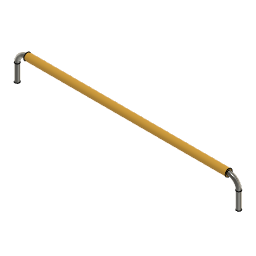
Full Piano (Autodesk Fusion 360 archive; units mm, degrees)
design "Yellow 13"
Autodesk Fusion 360 part; units mm, degrees
sketch "Sketch1" plane through (0, 0, 0) normal (0, 1, 0) x (1, 0, 0)
  line L0 (1.5, 0) -> (31.52, 0)
  line L1 (0, 1.5) -> (0, 4)
  line L2 (33.02, 1.5) -> (33.02, 4)
  arc A0 (0, 1.5) -> (1.5, 0) centre (1.5, 1.5) ccw
  arc A1 (31.52, 0) -> (33.02, 1.5) centre (31.52, 1.5) ccw
  point P0 (33.02, 0)
  dimension "d6" = 33.02
  dimension "d7" = 4
  dimension "d8" = 4
  dimension "d10" = 1.5
  dimension "d11" = 1.5
  constraint horizontal L0
  constraint perpendicular L0 L1
  constraint perpendicular L0 L2
  constraint coincident origin L0
  constraint coincident origin L1
  constraint tangent L1 A0
  constraint tangent L0 A0
  constraint coincident P0 L0
  constraint coincident P0 L2
  constraint tangent L0 A1
  constraint tangent L2 A1
  measures "d6" distance of origin P0
  measures "d7" distance of origin L1.end
  measures "d8" distance of P0 L2.end
  measures "d10" radius of A0
  measures "d11" radius of A1
pipe "Pipe1" add diameter 0.64 path "Sketch1" along L1 A0 L0 A1 L2 makes body 1
ref_plane "WorkPlane1" through (1.5, 0, 0) normal (1, 0, 0) x (0, 1, 0)
sketch "Sketch2" plane through (1.5, 0, 0) normal (1, 0, 0) x (0, 1, 0)
  circle A0 centre (0, 0) radius 0.52
  circle A1 centre (0, 0) radius 0.32
  dimension "d18" = 1.04
  dimension "d19" = 0.64
  constraint coincident A0.centre A1.centre
  constraint concentric A0 A1
  measures "d18" diameter of A0
  measures "d19" diameter of A1
ref_plane "WorkPlane2" through (31.52, 0, 0) normal (1, 0, 0) x (0, 1, 0)
extrude "Extrude1" add sketch "Sketch2" along normal up to surface (30.02 mm away) separate body makes body 2
equation "WireGauge = 0.64 mm"
equation "InsulationThickness = 0.4 mm"
equation "Length = 13"
equation "HoleSpacing = 2.54 mm"
equation "d6 = HoleSpacing * Length"
equation "d7 = ExtraLength"
equation "d8 = ExtraLength"
equation "ExtraLength = 4 mm"
equation "d10 = Arc"
equation "d11 = Arc"
equation "Arc = 1.5 mm"
equation "d15 = WireGauge"
equation "d18 = InsulationThickness + WireGauge"
equation "d19 = WireGauge"

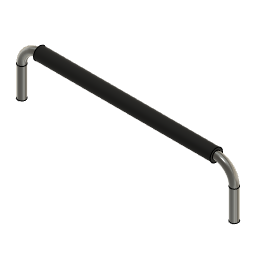
design "Black 8"
Autodesk Fusion 360 part; units mm, degrees
sketch "Sketch1" plane through (0, 0, 0) normal (0, 1, 0) x (1, 0, 0)
  line L0 (1.5, 0) -> (16.28, 0)
  line L1 (0, 1.5) -> (0, 4)
  line L2 (17.78, 1.5) -> (17.78, 4)
  arc A0 (0, 1.5) -> (1.5, 0) centre (1.5, 1.5) ccw
  arc A1 (16.28, 0) -> (17.78, 1.5) centre (16.28, 1.5) ccw
  point P0 (17.78, 0)
  dimension "d6" = 17.78
  dimension "d7" = 4
  dimension "d8" = 4
  dimension "d10" = 1.5
  dimension "d11" = 1.5
  constraint horizontal L0
  constraint perpendicular L0 L1
  constraint perpendicular L0 L2
  constraint coincident origin L0
  constraint coincident origin L1
  constraint tangent L1 A0
  constraint tangent L0 A0
  constraint coincident P0 L0
  constraint coincident P0 L2
  constraint tangent L0 A1
  constraint tangent L2 A1
  measures "d6" distance of origin P0
  measures "d7" distance of origin L1.end
  measures "d8" distance of P0 L2.end
  measures "d10" radius of A0
  measures "d11" radius of A1
pipe "Pipe1" add diameter 0.64 path "Sketch1" along L1 A0 L0 A1 L2 makes body 1
ref_plane "WorkPlane1" through (1.5, 0, 0) normal (1, 0, 0) x (0, 1, 0)
sketch "Sketch2" plane through (1.5, 0, 0) normal (1, 0, 0) x (0, 1, 0)
  circle A0 centre (0, 0) radius 0.52
  circle A1 centre (0, 0) radius 0.32
  dimension "d18" = 1.04
  dimension "d19" = 0.64
  constraint coincident A0.centre A1.centre
  constraint concentric A0 A1
  measures "d18" diameter of A0
  measures "d19" diameter of A1
ref_plane "WorkPlane2" through (16.28, 0, 0) normal (1, 0, 0) x (0, 1, 0)
extrude "Extrude1" add sketch "Sketch2" along normal up to surface (14.78 mm away) separate body makes body 2
equation "WireGauge = 0.64 mm"
equation "InsulationThickness = 0.4 mm"
equation "Length = 8"
equation "HoleSpacing = 2.54 mm"
equation "d6 = HoleSpacing * ( Length - 1 )"
equation "d7 = ExtraLength"
equation "d8 = ExtraLength"
equation "ExtraLength = 4 mm"
equation "d10 = Arc"
equation "d11 = Arc"
equation "Arc = 1.5 mm"
equation "d15 = WireGauge"
equation "d18 = InsulationThickness + WireGauge"
equation "d19 = WireGauge"

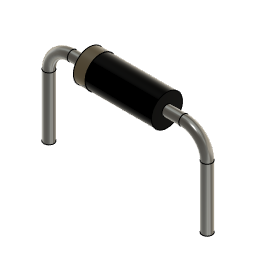
design "Diode 2"
Autodesk Fusion 360 part; units mm, degrees
sketch "Sketch1" plane through (0, 0, 0) normal (0, 1, 0) x (1, 0, 0)
  line L0 (1.5, 0) -> (8.66, 0)
  line L1 (0, 1.5) -> (0, 5.5)
  line L2 (10.16, 1.5) -> (10.16, 5.5)
  arc A0 (0, 1.5) -> (1.5, 0) centre (1.5, 1.5) ccw
  arc A1 (8.66, 0) -> (10.16, 1.5) centre (8.66, 1.5) ccw
  point P0 (10.16, 0)
  dimension "d6" = 10.16
  dimension "d7" = 5.5
  dimension "d8" = 5.5
  dimension "d10" = 1.5
  dimension "d11" = 1.5
  constraint horizontal L0
  constraint perpendicular L0 L1
  constraint perpendicular L0 L2
  constraint coincident origin L0
  constraint coincident origin L1
  constraint tangent L1 A0
  constraint tangent L0 A0
  constraint coincident P0 L0
  constraint coincident P0 L2
  constraint tangent L0 A1
  constraint tangent L2 A1
  measures "d6" distance of origin P0
  measures "d7" distance of origin L1.end
  measures "d8" distance of P0 L2.end
  measures "d10" radius of A0
  measures "d11" radius of A1
pipe "Pipe1" add diameter 0.64 path "Sketch1" along L1 A0 L0 A1 L2
ref_plane "WorkPlane1" through (1.5, 0, 0) normal (1, 0, 0) x (0, 1, 0)
sketch "Sketch2" plane through (1.5, 0, 0) normal (1, 0, 0) x (0, 1, 0)
  circle A0 centre (0, 0) radius 0.52
  circle A1 centre (0, 0) radius 0.32
  dimension "d18" = 1.04
  dimension "d19" = 0.64
  constraint coincident A0.centre A1.centre
  constraint concentric A0 A1
  measures "d18" diameter of A0
  measures "d19" diameter of A1
ref_plane "WorkPlane2" through (8.66, 0, 0) normal (1, 0, 0) x (0, 1, 0)
ref_plane "WorkPlane3" through (-0.32, 0, -3.8241) normal (-1, 0, 0) x (0, 1, 0)
ref_plane "WorkPlane4" through (10.48, 0, -1.931) normal (1, 0, 0) x (0, 1, 0)
ref_plane "WorkPlane5" through (5.08, 0, -3.8241) normal (-1, 0, 0) x (0, 1, 0)
sketch "Sketch3" plane through (5.08, 0, -2.3241) normal (-1, 0, 0) x (0, 1, 0)
  circle A0 centre (0, -2.3241) radius 0.32
  circle A1 centre (0, -2.3241) radius 1
  dimension "d27" = 2
  constraint concentric A0 A1
  measures "d27" diameter of A1
extrude "Extrude2" add sketch "Sketch3" along normal mid plane 5
sketch "Sketch4" plane through (2.58, 0, 0) normal (-1, 0, 0) x (0, -1, 0)
  circle A0 centre (0, 0) radius 0.32
  circle A1 centre (0, 0) radius 1
  circle A2 centre (0, 0) radius 1.01
  dimension "d30" = 0.01
  constraint coincident A0.centre A1.centre
  measures "d30" distance of A1 A2
extrude "Extrude3" add sketch "Sketch4" against normal blind 0.75 contours A2
equation "WireGauge = 0.64 mm"
equation "InsulationThickness = 0.4 mm"
equation "Length = 5"
equation "HoleSpacing = 2.54 mm"
equation "d6 = HoleSpacing * ( Length - 1 )"
equation "d7 = ExtraLength"
equation "d8 = ExtraLength"
equation "ExtraLength = 5.5 mm"
equation "d10 = Arc"
equation "d11 = Arc"
equation "Arc = 1.5 mm"
equation "d15 = WireGauge"
equation "d18 = InsulationThickness + WireGauge"
equation "d19 = WireGauge"

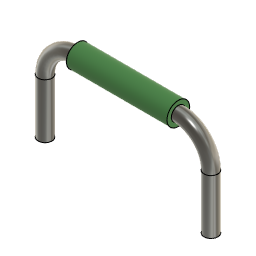
design "Green 4"
Autodesk Fusion 360 part; units mm, degrees
sketch "Sketch1" plane through (0, 0, 0) normal (0, 1, 0) x (1, 0, 0)
  line L0 (1.5, 0) -> (6.12, 0)
  line L1 (0, 1.5) -> (0, 4)
  line L2 (7.62, 1.5) -> (7.62, 4)
  arc A0 (0, 1.5) -> (1.5, 0) centre (1.5, 1.5) ccw
  arc A1 (6.12, 0) -> (7.62, 1.5) centre (6.12, 1.5) ccw
  point P0 (7.62, 0)
  dimension "d6" = 7.62
  dimension "d7" = 4
  dimension "d8" = 4
  dimension "d10" = 1.5
  dimension "d11" = 1.5
  constraint horizontal L0
  constraint perpendicular L0 L1
  constraint perpendicular L0 L2
  constraint coincident origin L0
  constraint coincident origin L1
  constraint tangent L1 A0
  constraint tangent L0 A0
  constraint coincident P0 L0
  constraint coincident P0 L2
  constraint tangent L0 A1
  constraint tangent L2 A1
  measures "d6" distance of origin P0
  measures "d7" distance of origin L1.end
  measures "d8" distance of P0 L2.end
  measures "d10" radius of A0
  measures "d11" radius of A1
pipe "Pipe1" add diameter 0.64 path "Sketch1" along L1 A0 L0 A1 L2 makes body 1
ref_plane "WorkPlane1" through (1.5, 0, 0) normal (1, 0, 0) x (0, 1, 0)
sketch "Sketch2" plane through (1.5, 0, 0) normal (1, 0, 0) x (0, 1, 0)
  circle A0 centre (0, 0) radius 0.52
  circle A1 centre (0, 0) radius 0.32
  dimension "d18" = 1.04
  dimension "d19" = 0.64
  constraint coincident A0.centre A1.centre
  constraint concentric A0 A1
  measures "d18" diameter of A0
  measures "d19" diameter of A1
ref_plane "WorkPlane2" through (6.12, 0, 0) normal (1, 0, 0) x (0, 1, 0)
extrude "Extrude1" add sketch "Sketch2" along normal up to surface (4.62 mm away) separate body makes body 2
equation "WireGauge = 0.64 mm"
equation "InsulationThickness = 0.4 mm"
equation "Length = 4"
equation "HoleSpacing = 2.54 mm"
equation "d6 = HoleSpacing * ( Length - 1 )"
equation "d7 = ExtraLength"
equation "d8 = ExtraLength"
equation "ExtraLength = 4 mm"
equation "d10 = Arc"
equation "d11 = Arc"
equation "Arc = 1.5 mm"
equation "d15 = WireGauge"
equation "d18 = InsulationThickness + WireGauge"
equation "d19 = WireGauge"

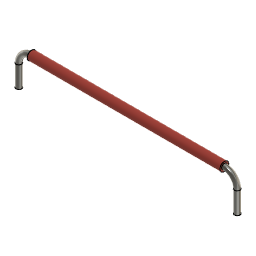
design "Red Diagonal"
Autodesk Fusion 360 part; units mm, degrees
sketch "Sketch1" plane through (0, 0, 0) normal (0, 1, 0) x (1, 0, 0)
  line L0 (1.5, 0) -> (24.0267, 0)
  line L1 (0, 1.5) -> (0, 4)
  line L2 (25.5267, 1.5) -> (25.5267, 4)
  arc A0 (0, 1.5) -> (1.5, 0) centre (1.5, 1.5) ccw
  arc A1 (24.0267, 0) -> (25.5267, 1.5) centre (24.0267, 1.5) ccw
  point P0 (25.5267, 0)
  dimension "d6" = 25.5267
  dimension "d7" = 4
  dimension "d8" = 4
  dimension "d10" = 1.5
  dimension "d11" = 1.5
  constraint horizontal L0
  constraint perpendicular L0 L1
  constraint perpendicular L0 L2
  constraint coincident origin L0
  constraint coincident origin L1
  constraint tangent L1 A0
  constraint tangent L0 A0
  constraint coincident P0 L0
  constraint coincident P0 L2
  constraint tangent L0 A1
  constraint tangent L2 A1
  measures "d6" distance of origin P0
  measures "d7" distance of origin L1.end
  measures "d8" distance of P0 L2.end
  measures "d10" radius of A0
  measures "d11" radius of A1
pipe "Pipe1" add diameter 0.64 path "Sketch1" along L1 A0 L0 A1 L2 makes body 1
ref_plane "WorkPlane1" through (1.5, 0, 0) normal (1, 0, 0) x (0, 1, 0)
sketch "Sketch2" plane through (1.5, 0, 0) normal (1, 0, 0) x (0, 1, 0)
  circle A0 centre (0, 0) radius 0.52
  circle A1 centre (0, 0) radius 0.32
  dimension "d18" = 1.04
  dimension "d19" = 0.64
  constraint coincident A0.centre A1.centre
  constraint concentric A0 A1
  measures "d18" diameter of A0
  measures "d19" diameter of A1
ref_plane "WorkPlane2" through (24.0267, 0, 0) normal (1, 0, 0) x (0, 1, 0)
extrude "Extrude1" add sketch "Sketch2" along normal up to surface (22.5267 mm away) separate body makes body 2
equation "WireGauge = 0.64 mm"
equation "InsulationThickness = 0.4 mm"
equation "Length = 4"
equation "HoleSpacing = 2.54 mm"
equation "d7 = ExtraLength"
equation "d8 = ExtraLength"
equation "ExtraLength = 4 mm"
equation "d10 = Arc"
equation "d11 = Arc"
equation "Arc = 1.5 mm"
equation "d15 = WireGauge"
equation "d18 = InsulationThickness + WireGauge"
equation "d19 = WireGauge"

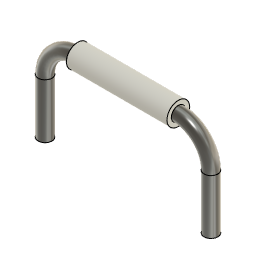
design "White 4"
Autodesk Fusion 360 part; units mm, degrees
sketch "Sketch1" plane through (0, 0, 0) normal (0, 1, 0) x (1, 0, 0)
  line L0 (1.5, 0) -> (6.12, 0)
  line L1 (0, 1.5) -> (0, 4)
  line L2 (7.62, 1.5) -> (7.62, 4)
  arc A0 (0, 1.5) -> (1.5, 0) centre (1.5, 1.5) ccw
  arc A1 (6.12, 0) -> (7.62, 1.5) centre (6.12, 1.5) ccw
  point P0 (7.62, 0)
  dimension "d6" = 7.62
  dimension "d7" = 4
  dimension "d8" = 4
  dimension "d10" = 1.5
  dimension "d11" = 1.5
  constraint horizontal L0
  constraint perpendicular L0 L1
  constraint perpendicular L0 L2
  constraint coincident origin L0
  constraint coincident origin L1
  constraint tangent L1 A0
  constraint tangent L0 A0
  constraint coincident P0 L0
  constraint coincident P0 L2
  constraint tangent L0 A1
  constraint tangent L2 A1
  measures "d6" distance of origin P0
  measures "d7" distance of origin L1.end
  measures "d8" distance of P0 L2.end
  measures "d10" radius of A0
  measures "d11" radius of A1
pipe "Pipe1" add diameter 0.64 path "Sketch1" along L1 A0 L0 A1 L2 makes body 1
ref_plane "WorkPlane1" through (1.5, 0, 0) normal (1, 0, 0) x (0, 1, 0)
sketch "Sketch2" plane through (1.5, 0, 0) normal (1, 0, 0) x (0, 1, 0)
  circle A0 centre (0, 0) radius 0.52
  circle A1 centre (0, 0) radius 0.32
  dimension "d18" = 1.04
  dimension "d19" = 0.64
  constraint coincident A0.centre A1.centre
  constraint concentric A0 A1
  measures "d18" diameter of A0
  measures "d19" diameter of A1
ref_plane "WorkPlane2" through (6.12, 0, 0) normal (1, 0, 0) x (0, 1, 0)
extrude "Extrude1" add sketch "Sketch2" along normal up to surface (4.62 mm away) separate body makes body 2
equation "WireGauge = 0.64 mm"
equation "InsulationThickness = 0.4 mm"
equation "Length = 4"
equation "HoleSpacing = 2.54 mm"
equation "d6 = HoleSpacing * ( Length - 1 )"
equation "d7 = ExtraLength"
equation "d8 = ExtraLength"
equation "ExtraLength = 4 mm"
equation "d10 = Arc"
equation "d11 = Arc"
equation "Arc = 1.5 mm"
equation "d15 = WireGauge"
equation "d18 = InsulationThickness + WireGauge"
equation "d19 = WireGauge"

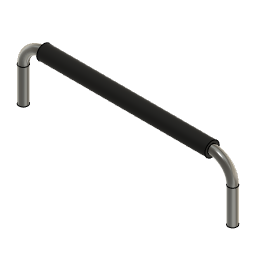
design "Black 7"
Autodesk Fusion 360 part; units mm, degrees
sketch "Sketch1" plane through (0, 0, 0) normal (0, 1, 0) x (1, 0, 0)
  line L0 (1.5, 0) -> (13.74, 0)
  line L1 (0, 1.5) -> (0, 4)
  line L2 (15.24, 1.5) -> (15.24, 4)
  arc A0 (0, 1.5) -> (1.5, 0) centre (1.5, 1.5) ccw
  arc A1 (13.74, 0) -> (15.24, 1.5) centre (13.74, 1.5) ccw
  point P0 (15.24, 0)
  dimension "d6" = 15.24
  dimension "d7" = 4
  dimension "d8" = 4
  dimension "d10" = 1.5
  dimension "d11" = 1.5
  constraint horizontal L0
  constraint perpendicular L0 L1
  constraint perpendicular L0 L2
  constraint coincident origin L0
  constraint coincident origin L1
  constraint tangent L1 A0
  constraint tangent L0 A0
  constraint coincident P0 L0
  constraint coincident P0 L2
  constraint tangent L0 A1
  constraint tangent L2 A1
  measures "d6" distance of origin P0
  measures "d7" distance of origin L1.end
  measures "d8" distance of P0 L2.end
  measures "d10" radius of A0
  measures "d11" radius of A1
pipe "Pipe1" add diameter 0.64 path "Sketch1" along L1 A0 L0 A1 L2 makes body 1
ref_plane "WorkPlane1" through (1.5, 0, 0) normal (1, 0, 0) x (0, 1, 0)
sketch "Sketch2" plane through (1.5, 0, 0) normal (1, 0, 0) x (0, 1, 0)
  circle A0 centre (0, 0) radius 0.52
  circle A1 centre (0, 0) radius 0.32
  dimension "d18" = 1.04
  dimension "d19" = 0.64
  constraint coincident A0.centre A1.centre
  constraint concentric A0 A1
  measures "d18" diameter of A0
  measures "d19" diameter of A1
ref_plane "WorkPlane2" through (13.74, 0, 0) normal (1, 0, 0) x (0, 1, 0)
extrude "Extrude1" add sketch "Sketch2" along normal up to surface (12.24 mm away) separate body makes body 2
equation "WireGauge = 0.64 mm"
equation "InsulationThickness = 0.4 mm"
equation "Length = 7"
equation "HoleSpacing = 2.54 mm"
equation "d6 = HoleSpacing * ( Length - 1 )"
equation "d7 = ExtraLength"
equation "d8 = ExtraLength"
equation "ExtraLength = 4 mm"
equation "d10 = Arc"
equation "d11 = Arc"
equation "Arc = 1.5 mm"
equation "d15 = WireGauge"
equation "d18 = InsulationThickness + WireGauge"
equation "d19 = WireGauge"

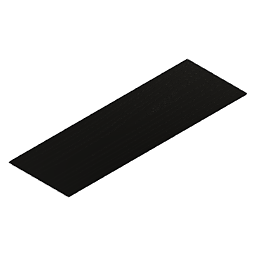
design "Piano Small Key"
Autodesk Fusion 360 part; units mm, degrees
sketch "Sketch1" plane through (0, 0, 0) normal (0, 0, 1) x (1, 0, 0)
  line L0 (0, 0) -> (152.4, 0)
  line L1 (152.4, 0) -> (152.4, 457.2)
  line L2 (152.4, 457.2) -> (0, 457.2)
  line L3 (0, 457.2) -> (0, 0)
  dimension "d4" = 152.4
  dimension "d5" = 457.2
  constraint horizontal L0
  constraint vertical L1
  constraint horizontal L2
  constraint vertical L3
  constraint coincident L0.start L3.end
  measures "d4" distance of L1.end L2.end
  measures "d5" distance of L0.start L2.end
extrude "Extrude1" add sketch "Sketch1" along normal blind 1
equation "SmallKeyWidth = 5.75 in"
equation "SmallKeyHeight = 18 in"
equation "d5 = SmallKeyHeight"

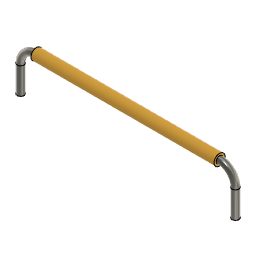
design "Yellow 8"
Autodesk Fusion 360 part; units mm, degrees
sketch "Sketch1" plane through (0, 0, 0) normal (0, 1, 0) x (1, 0, 0)
  line L0 (1.5, 0) -> (18.82, 0)
  line L1 (0, 1.5) -> (0, 4)
  line L2 (20.32, 1.5) -> (20.32, 4)
  arc A0 (0, 1.5) -> (1.5, 0) centre (1.5, 1.5) ccw
  arc A1 (18.82, 0) -> (20.32, 1.5) centre (18.82, 1.5) ccw
  point P0 (20.32, 0)
  dimension "d6" = 20.32
  dimension "d7" = 4
  dimension "d8" = 4
  dimension "d10" = 1.5
  dimension "d11" = 1.5
  constraint horizontal L0
  constraint perpendicular L0 L1
  constraint perpendicular L0 L2
  constraint coincident origin L0
  constraint coincident origin L1
  constraint tangent L1 A0
  constraint tangent L0 A0
  constraint coincident P0 L0
  constraint coincident P0 L2
  constraint tangent L0 A1
  constraint tangent L2 A1
  measures "d6" distance of origin P0
  measures "d7" distance of origin L1.end
  measures "d8" distance of P0 L2.end
  measures "d10" radius of A0
  measures "d11" radius of A1
pipe "Pipe1" add diameter 0.64 path "Sketch1" along L1 A0 L0 A1 L2 makes body 1
ref_plane "WorkPlane1" through (1.5, 0, 0) normal (1, 0, 0) x (0, 1, 0)
sketch "Sketch2" plane through (1.5, 0, 0) normal (1, 0, 0) x (0, 1, 0)
  circle A0 centre (0, 0) radius 0.52
  circle A1 centre (0, 0) radius 0.32
  dimension "d18" = 1.04
  dimension "d19" = 0.64
  constraint coincident A0.centre A1.centre
  constraint concentric A0 A1
  measures "d18" diameter of A0
  measures "d19" diameter of A1
ref_plane "WorkPlane2" through (18.82, 0, 0) normal (1, 0, 0) x (0, 1, 0)
extrude "Extrude1" add sketch "Sketch2" along normal up to surface (17.32 mm away) separate body makes body 2
equation "WireGauge = 0.64 mm"
equation "InsulationThickness = 0.4 mm"
equation "Length = 8"
equation "HoleSpacing = 2.54 mm"
equation "d6 = HoleSpacing * Length"
equation "d7 = ExtraLength"
equation "d8 = ExtraLength"
equation "ExtraLength = 4 mm"
equation "d10 = Arc"
equation "d11 = Arc"
equation "Arc = 1.5 mm"
equation "d15 = WireGauge"
equation "d18 = InsulationThickness + WireGauge"
equation "d19 = WireGauge"

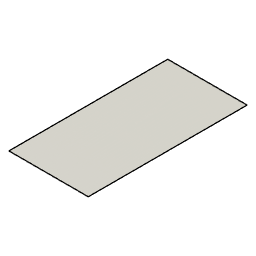
design "Piano Key Full"
Autodesk Fusion 360 part; units mm, degrees
sketch "Sketch1" plane through (0, 0, 0) normal (0, 0, 1) x (1, 0, 0)
  line L0 (0, 0) -> (304.8, 0)
  line L1 (304.8, 0) -> (304.8, 609.6)
  line L2 (304.8, 609.6) -> (0, 609.6)
  line L3 (0, 609.6) -> (0, 0)
  line L4 (0, 609.6) -> (146.05, 609.6)
  line L5 (0, 152.4) -> (0, 609.6)
  dimension "d1" = 304.8
  dimension "d2" = 609.6
  constraint horizontal L0
  constraint vertical L1
  constraint horizontal L2
  constraint vertical L3
  constraint coincident L0.start L3.end
  constraint horizontal L4
  constraint vertical L5
  measures "d1" distance of L1.end L2.end
  measures "d2" distance of L0.start L2.end
extrude "Extrude1" add sketch "Sketch1" along normal blind 1
equation "d1 = KeyWidth"
equation "d2 = KeyHeight"
equation "KeyWidth = 12 in"
equation "KeyHeight = 24 in"
equation "SmallKeyWidth = 5.75 in"
equation "SmallKeyHeight = 18 in"

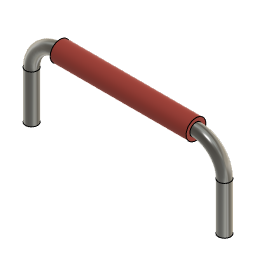
design "Red 5"
Autodesk Fusion 360 part; units mm, degrees
sketch "Sketch1" plane through (0, 0, 0) normal (0, 1, 0) x (1, 0, 0)
  line L0 (1.5, 0) -> (8.66, 0)
  line L1 (0, 1.5) -> (0, 4)
  line L2 (10.16, 1.5) -> (10.16, 4)
  arc A0 (0, 1.5) -> (1.5, 0) centre (1.5, 1.5) ccw
  arc A1 (8.66, 0) -> (10.16, 1.5) centre (8.66, 1.5) ccw
  point P0 (10.16, 0)
  dimension "d6" = 10.16
  dimension "d7" = 4
  dimension "d8" = 4
  dimension "d10" = 1.5
  dimension "d11" = 1.5
  constraint horizontal L0
  constraint perpendicular L0 L1
  constraint perpendicular L0 L2
  constraint coincident origin L0
  constraint coincident origin L1
  constraint tangent L1 A0
  constraint tangent L0 A0
  constraint coincident P0 L0
  constraint coincident P0 L2
  constraint tangent L0 A1
  constraint tangent L2 A1
  measures "d6" distance of origin P0
  measures "d7" distance of origin L1.end
  measures "d8" distance of P0 L2.end
  measures "d10" radius of A0
  measures "d11" radius of A1
pipe "Pipe1" add diameter 0.64 path "Sketch1" along L1 A0 L0 A1 L2 makes body 1
ref_plane "WorkPlane1" through (1.5, 0, 0) normal (1, 0, 0) x (0, 1, 0)
sketch "Sketch2" plane through (1.5, 0, 0) normal (1, 0, 0) x (0, 1, 0)
  circle A0 centre (0, 0) radius 0.52
  circle A1 centre (0, 0) radius 0.32
  dimension "d18" = 1.04
  dimension "d19" = 0.64
  constraint coincident A0.centre A1.centre
  constraint concentric A0 A1
  measures "d18" diameter of A0
  measures "d19" diameter of A1
ref_plane "WorkPlane2" through (8.66, 0, 0) normal (1, 0, 0) x (0, 1, 0)
extrude "Extrude1" add sketch "Sketch2" along normal up to surface (7.16 mm away) separate body makes body 2
equation "WireGauge = 0.64 mm"
equation "InsulationThickness = 0.4 mm"
equation "Length = 5"
equation "HoleSpacing = 2.54 mm"
equation "d6 = HoleSpacing * ( Length - 1 )"
equation "d7 = ExtraLength"
equation "d8 = ExtraLength"
equation "ExtraLength = 4 mm"
equation "d10 = Arc"
equation "d11 = Arc"
equation "Arc = 1.5 mm"
equation "d15 = WireGauge"
equation "d18 = InsulationThickness + WireGauge"
equation "d19 = WireGauge"

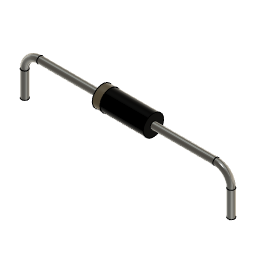
design "Diode 1"
Autodesk Fusion 360 part; units mm, degrees
sketch "Sketch1" plane through (0, 0, 0) normal (0, 1, 0) x (1, 0, 0)
  line L0 (1.5, 0) -> (18.82, 0)
  line L1 (0, 1.5) -> (0, 4)
  line L2 (20.32, 1.5) -> (20.32, 4)
  arc A0 (0, 1.5) -> (1.5, 0) centre (1.5, 1.5) ccw
  arc A1 (18.82, 0) -> (20.32, 1.5) centre (18.82, 1.5) ccw
  point P0 (20.32, 0)
  dimension "d6" = 20.32
  dimension "d7" = 4
  dimension "d8" = 4
  dimension "d10" = 1.5
  dimension "d11" = 1.5
  constraint horizontal L0
  constraint perpendicular L0 L1
  constraint perpendicular L0 L2
  constraint coincident origin L0
  constraint coincident origin L1
  constraint tangent L1 A0
  constraint tangent L0 A0
  constraint coincident P0 L0
  constraint coincident P0 L2
  constraint tangent L0 A1
  constraint tangent L2 A1
  measures "d6" distance of origin P0
  measures "d7" distance of origin L1.end
  measures "d8" distance of P0 L2.end
  measures "d10" radius of A0
  measures "d11" radius of A1
pipe "Pipe1" add diameter 0.64 path "Sketch1" along L1 A0 L0 A1 L2
ref_plane "WorkPlane1" through (1.5, 0, 0) normal (1, 0, 0) x (0, 1, 0)
sketch "Sketch2" plane through (1.5, 0, 0) normal (1, 0, 0) x (0, 1, 0)
  circle A0 centre (0, 0) radius 0.52
  circle A1 centre (0, 0) radius 0.32
  dimension "d18" = 1.04
  dimension "d19" = 0.64
  constraint coincident A0.centre A1.centre
  constraint concentric A0 A1
  measures "d18" diameter of A0
  measures "d19" diameter of A1
ref_plane "WorkPlane2" through (18.82, 0, 0) normal (1, 0, 0) x (0, 1, 0)
ref_plane "WorkPlane3" through (-0.32, 0, -2.3241) normal (-1, 0, 0) x (0, 1, 0)
ref_plane "WorkPlane4" through (20.64, 0, -1.931) normal (1, 0, 0) x (0, 1, 0)
ref_plane "WorkPlane5" through (10.16, 0, -2.3241) normal (-1, 0, 0) x (0, 1, 0)
sketch "Sketch3" plane through (10.16, 0, -2.3241) normal (-1, 0, 0) x (0, 1, 0)
  circle A0 centre (0, -2.3241) radius 0.32
  circle A1 centre (0, -2.3241) radius 1
  dimension "d27" = 2
  constraint concentric A0 A1
  measures "d27" diameter of A1
extrude "Extrude2" add sketch "Sketch3" along normal mid plane 5
sketch "Sketch4" plane through (7.66, 0, 0) normal (-1, 0, 0) x (0, -1, 0)
  circle A0 centre (0, 0) radius 0.32
  circle A1 centre (0, 0) radius 1
  circle A2 centre (0, 0) radius 1.01
  dimension "d30" = 0.01
  constraint coincident A0.centre A1.centre
  measures "d30" distance of A1 A2
extrude "Extrude3" add sketch "Sketch4" against normal blind 0.75 contours A2
equation "WireGauge = 0.64 mm"
equation "InsulationThickness = 0.4 mm"
equation "Length = 9"
equation "HoleSpacing = 2.54 mm"
equation "d6 = HoleSpacing * ( Length - 1 )"
equation "d7 = ExtraLength"
equation "d8 = ExtraLength"
equation "ExtraLength = 4 mm"
equation "d10 = Arc"
equation "d11 = Arc"
equation "Arc = 1.5 mm"
equation "d15 = WireGauge"
equation "d18 = InsulationThickness + WireGauge"
equation "d19 = WireGauge"

design "Blue 4 - Diagonal"
Autodesk Fusion 360 part; units mm, degrees
sketch "Sketch1" plane through (0, 0, 0) normal (0, 1, 0) x (1, 0, 0)
  line L0 (1.5, 0) -> (9.2763, 0)
  line L1 (0, 1.5) -> (0, 4)
  line L2 (10.7763, 1.5) -> (10.7763, 4)
  arc A0 (0, 1.5) -> (1.5, 0) centre (1.5, 1.5) ccw
  arc A1 (9.2763, 0) -> (10.7763, 1.5) centre (9.2763, 1.5) ccw
  point P0 (10.7763, 0)
  dimension "d6" = 10.7763
  dimension "d7" = 4
  dimension "d8" = 4
  dimension "d10" = 1.5
  dimension "d11" = 1.5
  constraint horizontal L0
  constraint perpendicular L0 L1
  constraint perpendicular L0 L2
  constraint coincident origin L0
  constraint coincident origin L1
  constraint tangent L1 A0
  constraint tangent L0 A0
  constraint coincident P0 L0
  constraint coincident P0 L2
  constraint tangent L0 A1
  constraint tangent L2 A1
  measures "d6" distance of origin P0
  measures "d7" distance of origin L1.end
  measures "d8" distance of P0 L2.end
  measures "d10" radius of A0
  measures "d11" radius of A1
pipe "Pipe1" add diameter 0.64 path "Sketch1" along L1 A0 L0 A1 L2 makes body 1
ref_plane "WorkPlane1" through (1.5, 0, 0) normal (1, 0, 0) x (0, 1, 0)
sketch "Sketch2" plane through (1.5, 0, 0) normal (1, 0, 0) x (0, 1, 0)
  circle A0 centre (0, 0) radius 0.52
  circle A1 centre (0, 0) radius 0.32
  dimension "d18" = 1.04
  dimension "d19" = 0.64
  constraint coincident A0.centre A1.centre
  constraint concentric A0 A1
  measures "d18" diameter of A0
  measures "d19" diameter of A1
ref_plane "WorkPlane2" through (9.2763, 0, 0) normal (1, 0, 0) x (0, 1, 0)
extrude "Extrude1" add sketch "Sketch2" along normal up to surface (7.7763 mm away) separate body makes body 2
equation "WireGauge = 0.64 mm"
equation "InsulationThickness = 0.4 mm"
equation "Length = 4"
equation "HoleSpacing = 2.54 mm"
equation "d6 = HoleSpacing * ( Length - 1 ) * 1.4142135623730951"
equation "d7 = ExtraLength"
equation "d8 = ExtraLength"
equation "ExtraLength = 4 mm"
equation "d10 = Arc"
equation "d11 = Arc"
equation "Arc = 1.5 mm"
equation "d15 = WireGauge"
equation "d18 = InsulationThickness + WireGauge"
equation "d19 = WireGauge"

design "Green 5"
Autodesk Fusion 360 part; units mm, degrees
sketch "Sketch1" plane through (0, 0, 0) normal (0, 1, 0) x (1, 0, 0)
  line L0 (1.5, 0) -> (8.66, 0)
  line L1 (0, 1.5) -> (0, 4)
  line L2 (10.16, 1.5) -> (10.16, 4)
  arc A0 (0, 1.5) -> (1.5, 0) centre (1.5, 1.5) ccw
  arc A1 (8.66, 0) -> (10.16, 1.5) centre (8.66, 1.5) ccw
  point P0 (10.16, 0)
  dimension "d6" = 10.16
  dimension "d7" = 4
  dimension "d8" = 4
  dimension "d10" = 1.5
  dimension "d11" = 1.5
  constraint horizontal L0
  constraint perpendicular L0 L1
  constraint perpendicular L0 L2
  constraint coincident origin L0
  constraint coincident origin L1
  constraint tangent L1 A0
  constraint tangent L0 A0
  constraint coincident P0 L0
  constraint coincident P0 L2
  constraint tangent L0 A1
  constraint tangent L2 A1
  measures "d6" distance of origin P0
  measures "d7" distance of origin L1.end
  measures "d8" distance of P0 L2.end
  measures "d10" radius of A0
  measures "d11" radius of A1
pipe "Pipe1" add diameter 0.64 path "Sketch1" along L1 A0 L0 A1 L2 makes body 1
ref_plane "WorkPlane1" through (1.5, 0, 0) normal (1, 0, 0) x (0, 1, 0)
sketch "Sketch2" plane through (1.5, 0, 0) normal (1, 0, 0) x (0, 1, 0)
  circle A0 centre (0, 0) radius 0.52
  circle A1 centre (0, 0) radius 0.32
  dimension "d18" = 1.04
  dimension "d19" = 0.64
  constraint coincident A0.centre A1.centre
  constraint concentric A0 A1
  measures "d18" diameter of A0
  measures "d19" diameter of A1
ref_plane "WorkPlane2" through (8.66, 0, 0) normal (1, 0, 0) x (0, 1, 0)
extrude "Extrude1" add sketch "Sketch2" along normal up to surface (7.16 mm away) separate body makes body 2
equation "WireGauge = 0.64 mm"
equation "InsulationThickness = 0.4 mm"
equation "Length = 5"
equation "HoleSpacing = 2.54 mm"
equation "d6 = HoleSpacing * ( Length - 1 )"
equation "d7 = ExtraLength"
equation "d8 = ExtraLength"
equation "ExtraLength = 4 mm"
equation "d10 = Arc"
equation "d11 = Arc"
equation "Arc = 1.5 mm"
equation "d15 = WireGauge"
equation "d18 = InsulationThickness + WireGauge"
equation "d19 = WireGauge"

design "Yellow 6"
Autodesk Fusion 360 part; units mm, degrees
sketch "Sketch1" plane through (0, 0, 0) normal (0, 1, 0) x (1, 0, 0)
  line L0 (1.5, 0) -> (11.2, 0)
  line L1 (0, 1.5) -> (0, 4)
  line L2 (12.7, 1.5) -> (12.7, 4)
  arc A0 (0, 1.5) -> (1.5, 0) centre (1.5, 1.5) ccw
  arc A1 (11.2, 0) -> (12.7, 1.5) centre (11.2, 1.5) ccw
  point P0 (12.7, 0)
  dimension "d6" = 12.7
  dimension "d7" = 4
  dimension "d8" = 4
  dimension "d10" = 1.5
  dimension "d11" = 1.5
  constraint horizontal L0
  constraint perpendicular L0 L1
  constraint perpendicular L0 L2
  constraint coincident origin L0
  constraint coincident origin L1
  constraint tangent L1 A0
  constraint tangent L0 A0
  constraint coincident P0 L0
  constraint coincident P0 L2
  constraint tangent L0 A1
  constraint tangent L2 A1
  measures "d6" distance of origin P0
  measures "d7" distance of origin L1.end
  measures "d8" distance of P0 L2.end
  measures "d10" radius of A0
  measures "d11" radius of A1
pipe "Pipe1" add diameter 0.64 path "Sketch1" along L1 A0 L0 A1 L2 makes body 1
ref_plane "WorkPlane1" through (1.5, 0, 0) normal (1, 0, 0) x (0, 1, 0)
sketch "Sketch2" plane through (1.5, 0, 0) normal (1, 0, 0) x (0, 1, 0)
  circle A0 centre (0, 0) radius 0.52
  circle A1 centre (0, 0) radius 0.32
  dimension "d18" = 1.04
  dimension "d19" = 0.64
  constraint coincident A0.centre A1.centre
  constraint concentric A0 A1
  measures "d18" diameter of A0
  measures "d19" diameter of A1
ref_plane "WorkPlane2" through (11.2, 0, 0) normal (1, 0, 0) x (0, 1, 0)
extrude "Extrude1" add sketch "Sketch2" along normal up to surface (9.7 mm away) separate body makes body 2
equation "WireGauge = 0.64 mm"
equation "InsulationThickness = 0.4 mm"
equation "Length = 6"
equation "HoleSpacing = 2.54 mm"
equation "d6 = HoleSpacing * ( Length - 1 )"
equation "d7 = ExtraLength"
equation "d8 = ExtraLength"
equation "ExtraLength = 4 mm"
equation "d10 = Arc"
equation "d11 = Arc"
equation "Arc = 1.5 mm"
equation "d15 = WireGauge"
equation "d18 = InsulationThickness + WireGauge"
equation "d19 = WireGauge"

design "Red 4"
Autodesk Fusion 360 part; units mm, degrees
sketch "Sketch1" plane through (0, 0, 0) normal (0, 1, 0) x (1, 0, 0)
  line L0 (1.5, 0) -> (6.12, 0)
  line L1 (0, 1.5) -> (0, 4)
  line L2 (7.62, 1.5) -> (7.62, 4)
  arc A0 (0, 1.5) -> (1.5, 0) centre (1.5, 1.5) ccw
  arc A1 (6.12, 0) -> (7.62, 1.5) centre (6.12, 1.5) ccw
  point P0 (7.62, 0)
  dimension "d6" = 7.62
  dimension "d7" = 4
  dimension "d8" = 4
  dimension "d10" = 1.5
  dimension "d11" = 1.5
  constraint horizontal L0
  constraint perpendicular L0 L1
  constraint perpendicular L0 L2
  constraint coincident origin L0
  constraint coincident origin L1
  constraint tangent L1 A0
  constraint tangent L0 A0
  constraint coincident P0 L0
  constraint coincident P0 L2
  constraint tangent L0 A1
  constraint tangent L2 A1
  measures "d6" distance of origin P0
  measures "d7" distance of origin L1.end
  measures "d8" distance of P0 L2.end
  measures "d10" radius of A0
  measures "d11" radius of A1
pipe "Pipe1" add diameter 0.64 path "Sketch1" along L1 A0 L0 A1 L2 makes body 1
ref_plane "WorkPlane1" through (1.5, 0, 0) normal (1, 0, 0) x (0, 1, 0)
sketch "Sketch2" plane through (1.5, 0, 0) normal (1, 0, 0) x (0, 1, 0)
  circle A0 centre (0, 0) radius 0.52
  circle A1 centre (0, 0) radius 0.32
  dimension "d18" = 1.04
  dimension "d19" = 0.64
  constraint coincident A0.centre A1.centre
  constraint concentric A0 A1
  measures "d18" diameter of A0
  measures "d19" diameter of A1
ref_plane "WorkPlane2" through (6.12, 0, 0) normal (1, 0, 0) x (0, 1, 0)
extrude "Extrude1" add sketch "Sketch2" along normal up to surface (4.62 mm away) separate body makes body 2
equation "WireGauge = 0.64 mm"
equation "InsulationThickness = 0.4 mm"
equation "Length = 4"
equation "HoleSpacing = 2.54 mm"
equation "d6 = HoleSpacing * ( Length - 1 )"
equation "d7 = ExtraLength"
equation "d8 = ExtraLength"
equation "ExtraLength = 4 mm"
equation "d10 = Arc"
equation "d11 = Arc"
equation "Arc = 1.5 mm"
equation "d15 = WireGauge"
equation "d18 = InsulationThickness + WireGauge"
equation "d19 = WireGauge"

design "Red 12"
Autodesk Fusion 360 part; units mm, degrees
sketch "Sketch1" plane through (0, 0, 0) normal (0, 1, 0) x (1, 0, 0)
  line L0 (1.5, 0) -> (26.44, 0)
  line L1 (0, 1.5) -> (0, 4)
  line L2 (27.94, 1.5) -> (27.94, 4)
  arc A0 (0, 1.5) -> (1.5, 0) centre (1.5, 1.5) ccw
  arc A1 (26.44, 0) -> (27.94, 1.5) centre (26.44, 1.5) ccw
  point P0 (27.94, 0)
  dimension "d6" = 27.94
  dimension "d7" = 4
  dimension "d8" = 4
  dimension "d10" = 1.5
  dimension "d11" = 1.5
  constraint horizontal L0
  constraint perpendicular L0 L1
  constraint perpendicular L0 L2
  constraint coincident origin L0
  constraint coincident origin L1
  constraint tangent L1 A0
  constraint tangent L0 A0
  constraint coincident P0 L0
  constraint coincident P0 L2
  constraint tangent L0 A1
  constraint tangent L2 A1
  measures "d6" distance of origin P0
  measures "d7" distance of origin L1.end
  measures "d8" distance of P0 L2.end
  measures "d10" radius of A0
  measures "d11" radius of A1
pipe "Pipe1" add diameter 0.64 path "Sketch1" along L1 A0 L0 A1 L2 makes body 1
ref_plane "WorkPlane1" through (1.5, 0, 0) normal (1, 0, 0) x (0, 1, 0)
sketch "Sketch2" plane through (1.5, 0, 0) normal (1, 0, 0) x (0, 1, 0)
  circle A0 centre (0, 0) radius 0.52
  circle A1 centre (0, 0) radius 0.32
  dimension "d18" = 1.04
  dimension "d19" = 0.64
  constraint coincident A0.centre A1.centre
  constraint concentric A0 A1
  measures "d18" diameter of A0
  measures "d19" diameter of A1
ref_plane "WorkPlane2" through (26.44, 0, 0) normal (1, 0, 0) x (0, 1, 0)
extrude "Extrude1" add sketch "Sketch2" along normal up to surface (24.94 mm away) separate body makes body 2
equation "WireGauge = 0.64 mm"
equation "InsulationThickness = 0.4 mm"
equation "Length = 12"
equation "HoleSpacing = 2.54 mm"
equation "d6 = HoleSpacing * ( Length - 1 )"
equation "d7 = ExtraLength"
equation "d8 = ExtraLength"
equation "ExtraLength = 4 mm"
equation "d10 = Arc"
equation "d11 = Arc"
equation "Arc = 1.5 mm"
equation "d15 = WireGauge"
equation "d18 = InsulationThickness + WireGauge"
equation "d19 = WireGauge"
